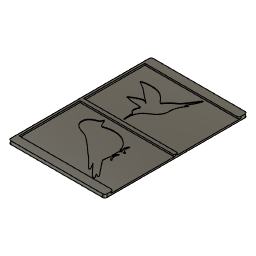
Wing Span - Lid (Autodesk Fusion 360 design; units mm, degrees)
Autodesk Fusion 360 part; units mm, degrees
note: some values were not read from the file. Set by a fixed rule: which sketch regions a step uses.
(part 1 of 2)
sketch "Skizze1" plane through (0, 0, 0) normal (0, 0, 1) x (1, 0, 0)
  line L0 (0, 0) -> (91.5, 0)
  line L1 (91.5, 0) -> (91.5, 135.5)
  line L2 (91.5, 135.5) -> (0, 135.5)
  line L3 (0, 135.5) -> (0, 0)
  line L4 (0, 0) -> (7, 0)
  line L5 (7, 0) -> (7, 7)
  line L6 (7, 7) -> (0, 7)
  line L7 (0, 7) -> (0, 0)
  line L8 (91.5, 0) -> (84.5, 0)
  line L9 (84.5, 0) -> (84.5, 7)
  line L10 (84.5, 7) -> (91.5, 7)
  line L11 (91.5, 7) -> (91.5, 0)
  line L12 (0, 135.5) -> (7, 135.5)
  line L13 (7, 135.5) -> (7, 128.5)
  line L14 (7, 128.5) -> (0, 128.5)
  line L15 (0, 128.5) -> (0, 135.5)
  line L16 (91.5, 135.5) -> (84.5, 135.5)
  line L17 (84.5, 135.5) -> (84.5, 128.5)
  line L18 (84.5, 128.5) -> (91.5, 128.5)
  line L19 (91.5, 128.5) -> (91.5, 135.5)
  circle A0 centre (3.5, 3.5) radius 2.675
  circle A1 centre (88, 3.5) radius 2.675
  circle A2 centre (88, 132) radius 2.675
  circle A3 centre (3.5, 132) radius 2.675
  dimension "d1" = 91.5
  dimension "d2" = 135.5
  dimension "d3" = 7
  dimension "d4" = 7
  dimension "d5" = 7
  dimension "d6" = 7
  dimension "d7" = 7
  dimension "d8" = 7
  dimension "d9" = 7
  dimension "d10" = 7
  dimension "d11" = 5.35
  dimension "d12" = 3.5
  dimension "d13" = 3.5
  dimension "d14" = 5.35
  dimension "d15" = 3.5
  dimension "d16" = 3.5
  dimension "d17" = 5.35
  dimension "d18" = 3.5
  dimension "d19" = 3.5
  dimension "d20" = 5.35
  dimension "d21" = 3.5
  dimension "d22" = 3.5
  constraint horizontal L0
  constraint vertical L1
  constraint horizontal L2
  constraint vertical L3
  constraint coincident L0.start L3.end
  constraint horizontal L4
  constraint vertical L5
  constraint horizontal L6
  constraint vertical L7
  constraint horizontal L8
  constraint vertical L9
  constraint horizontal L10
  constraint vertical L11
  constraint horizontal L12
  constraint vertical L13
  constraint horizontal L14
  constraint vertical L15
  constraint horizontal L16
  constraint vertical L17
  constraint horizontal L18
  constraint vertical L19
  measures "d1" distance of L0.start L0.end
  measures "d2" distance of L0.start L2.end
  measures "d3" distance of L0.start L4.end
  measures "d4" distance of L0.start L6.end
  measures "d5" distance of L0.end L8.end
  measures "d6" distance of L0.end L10.end
  measures "d7" distance of L2.end L12.end
  measures "d8" distance of L2.end L14.end
  measures "d9" distance of L1.end L16.end
  measures "d10" distance of L1.end L18.end
  measures "d11" diameter of A0
  measures "d12" distance of L4 A0.centre
  measures "d13" distance of L7 A0.centre
  measures "d14" diameter of A1
  measures "d15" distance of L11 A1.centre
  measures "d16" distance of L10 A1.centre
  measures "d17" diameter of A2
  measures "d18" distance of L19 A2.centre
  measures "d19" distance of L2 A2.centre
  measures "d20" diameter of A3
  measures "d21" distance of L12 A3.centre
  measures "d22" distance of L13 A3.centre
extrude "Extrusion6" add sketch "Skizze1" along normal blind 3 contours L0 L3 L4 L5 L6 L7 | L0 L1 L2 L3 L5 L6 L9 L10 L13 L14 L17 L18 | L0 L1 L8 L9 L10 L11 | L2 L3 L12 L13 L14 L15 | L1 L2 L16 L17 L18 L19 | A0 | A1 | A2 | A3 picked at (3.433366, 0.277493) picked at (58.666667, 47.5) picked at (87.933366, 0.277493) picked at (3.433366, 128.777493) picked at (88.066634, 128.777493) picked at (2.696636, 4.326095) picked at (88.803364, 3.621088) picked at (88.700923, 133.066531) picked at (1.893588, 131.564999)
extrude "Extrusion7" cut sketch "Skizze1" along normal blind 1.2 contours A0 | A1 | A2 | A3 picked at (2.696636, 4.326095) picked at (88.803364, 3.621088) picked at (88.700923, 133.066531) picked at (1.893588, 131.564999)
sketch "Skizze6" plane through (0, 0, 3) normal (0, 0, 1) x (-1, 0, 0)
  line L0 (-91.5, 0) -> (-91.5, -135.5)
  line L1 (-91.5, -135.5) -> (0, -135.5)
  line L2 (0, -135.5) -> (0, 0)
  line L3 (0, 0) -> (-91.5, 0)
  line L4 (-2, -8) -> (-91.5, -8)
  line L5 (-91.5, -8) -> (-91.5, -66)
  line L6 (-91.5, -66) -> (-2, -66)
  line L7 (-2, -66) -> (-2, -8)
  line L8 (-2, -69.499999) -> (-91.5, -69.499999)
  line L9 (-91.5, -69.499999) -> (-91.5, -127.5)
  line L10 (-91.5, -127.5) -> (-2, -127.5)
  line L11 (-2, -127.5) -> (-2, -69.499999)
  dimension "d51" = 89.5
  dimension "d52" = 58
  dimension "d53" = 2
  dimension "d54" = 8
  dimension "d55" = 2
  dimension "d56" = 58
  dimension "d57" = 8
  dimension "d58" = 89.5
  constraint horizontal L4
  constraint vertical L5
  constraint horizontal L6
  constraint vertical L7
  constraint horizontal L8
  constraint vertical L9
  constraint horizontal L10
  constraint vertical L11
  measures "d51" distance of L4.start L4.end
  measures "d52" distance of L4.start L6.end
  measures "d53" distance of L2 L7
  measures "d54" distance of L3 L4
  measures "d55" distance of L2 L11
  measures "d56" distance of L8 L10
  measures "d57" distance of L1 L10
  measures "d58" distance of L9 L11
extrude "Extrusion9" cut sketch "Skizze6" against normal blind 1.5 contours L0 L4 L5 L6 L7 | L0 L8 L9 L10 L11 picked at (-61.666667, -27.333333) picked at (-61.666667, -88.833333)
fillet "Abrundung3" radius 2 2 edges at (0, 0, 1.5) (0, 135.5, 1.5)
fillet "Abrundung4" radius 1 1 edges at (91.5, 66, 2.25)
fillet "Abrundung5" radius 1 1 edges at (91.5, 69.499999, 2.25)
fillet "Abrundung6" radius 2 1 edges at (91.5, 8, 2.25)
fillet "Abrundung7" radius 2 1 edges at (91.5, 127.5, 2.25)
fillet "Abrundung8" radius 2 2 edges at (91.5, 135.5, 1.5) (91.5, 0, 1.5)
sketch "Skizze7" plane through (0, 0, 1.5) normal (0, 0, 1) x (-1, 0, 0)
  line L0 (-2, -66) -> (-2, -8)
  line L1 (-2, -8) -> (-89.5, -8)
  arc A0 (-91.5, -6) -> (-89.5, -8) centre (-89.5, -6) ccw
  line L2 (-91.5, -6) -> (-91.5, -67)
  arc A1 (-90.5, -66) -> (-91.5, -67) centre (-90.5, -67) ccw
  line L3 (-90.5, -66) -> (-2, -66)
  spline S0 degree 3 poles (-30.411065, -58.609692) (-28.836348, -62.212151) (-28.526911, -62.854914) (-28.162708, -62.873627) knots 0 0 0 0 1 1 1 1
  spline S1 degree 3 poles (-28.162708, -62.873627) (-28.080965, -62.877743) (-27.963864, -62.847698) (-27.869518, -62.680787) knots 0 0 0 0 1 1 1 1
  spline S2 degree 3 poles (-27.869518, -62.680787) (-27.684016, -62.352588) (-27.563036, -62.031554) (-27.446005, -61.720969) knots 0 0 0 0 1 1 1 1
  spline S3 degree 3 poles (-27.446005, -61.720969) (-27.205823, -61.083809) (-26.998358, -60.533474) (-26.308111, -60.053195) knots 0 0 0 0 1 1 1 1
  spline S4 degree 3 poles (-26.308111, -60.053195) (-25.982101, -59.826301) (-25.405463, -59.594364) (-24.737778, -59.325714) knots 0 0 0 0 1 1 1 1
  spline S5 degree 3 poles (-24.737778, -59.325714) (-22.624632, -58.475447) (-19.431234, -57.190489) (-18.33478, -53.917152) knots 0 0 0 0 1 1 1 1
  spline S6 degree 3 poles (-18.33478, -53.917152) (-18.152793, -53.372845) (-18.035865, -52.81678) (-17.987487, -52.263824) knots 0 0 0 0 1 1 1 1
  spline S7 degree 3 poles (-17.987487, -52.263824) (-17.808073, -50.213115) (-18.547131, -48.264464) (-20.124662, -46.628865) knots 0 0 0 0 1 1 1 1
  spline S8 degree 3 poles (-20.124662, -46.628865) (-21.885668, -44.80306) (-24.550983, -43.48011) (-28.046934, -42.69664) knots 0 0 0 0 1 1 1 1
  spline S9 degree 3 poles (-28.046934, -42.69664) (-32.434766, -41.713249) (-40.268695, -34.518616) (-44.949472, -30.220073) knots 0 0 0 0 1 1 1 1
  spline S10 degree 3 poles (-44.949472, -30.220073) (-46.538387, -28.760833) (-47.793338, -27.608143) (-48.426302, -27.148487) knots 0 0 0 0 1 1 1 1
  spline S11 degree 3 poles (-48.426302, -27.148487) (-50.763295, -25.450827) (-53.762076, -22.368466) (-56.171671, -19.891637) knots 0 0 0 0 1 1 1 1
  spline S12 degree 3 poles (-56.171671, -19.891637) (-58.950819, -17.035183) (-60.429083, -15.544488) (-61.031372, -15.547429) knots 0 0 0 0 1 1 1 1
  spline S13 degree 3 poles (-61.031372, -15.547429) (-61.150111, -15.547999) (-61.224441, -15.599828) (-61.265834, -15.643243) knots 0 0 0 0 1 1 1 1
  spline S14 degree 3 poles (-61.265834, -15.643243) (-61.323003, -15.703148) (-61.356462, -15.785022) (-61.365362, -15.886746) knots 0 0 0 0 1 1 1 1
  spline S15 degree 3 poles (-61.365362, -15.886746) (-61.437672, -16.713253) (-59.650855, -19.65266) (-57.870181, -22.384839) knots 0 0 0 0 1 1 1 1
  spline S16 degree 3 poles (-57.870181, -22.384839) (-59.546777, -20.484485) (-61.836065, -18.04111) (-64.07326, -15.653713) knots 0 0 0 0 1 1 1 1
  spline S17 degree 3 poles (-64.07326, -15.653713) (-64.765743, -14.914723) (-65.44634, -14.188238) (-66.091815, -13.495845) knots 0 0 0 0 1 1 1 1
  spline S18 degree 3 poles (-66.091815, -13.495845) (-68.098082, -11.343941) (-69.849858, -10.110189) (-70.554899, -10.352979) knots 0 0 0 0 1 1 1 1
  spline S19 degree 3 poles (-70.554899, -10.352979) (-70.7336, -10.414559) (-70.842148, -10.562693) (-70.860284, -10.769989) knots 0 0 0 0 1 1 1 1
  spline S20 degree 3 poles (-70.860284, -10.769989) (-70.909057, -11.327464) (-70.309448, -12.235853) (-69.797711, -12.899855) knots 0 0 0 0 1 1 1 1
  spline S21 degree 3 poles (-69.797711, -12.899855) (-68.87248, -14.100238) (-68.549162, -14.7867) (-68.552585, -15.037768) knots 0 0 0 0 1 1 1 1
  spline S22 degree 3 poles (-68.552585, -15.037768) (-68.62865, -15.030438) (-68.844737, -14.948986) (-69.247923, -14.618512) knots 0 0 0 0 1 1 1 1
  spline S23 degree 3 poles (-69.247923, -14.618512) (-70.158248, -13.872096) (-70.957131, -13.534144) (-71.384918, -13.714199) knots 0 0 0 0 1 1 1 1
  spline S24 degree 3 poles (-71.384918, -13.714199) (-71.554173, -13.785372) (-71.656843, -13.931829) (-71.673866, -14.12641) knots 0 0 0 0 1 1 1 1
  spline S25 degree 3 poles (-71.673866, -14.12641) (-71.709714, -14.53615) (-71.359214, -15.158565) (-70.687885, -15.879183) knots 0 0 0 0 1 1 1 1
  spline S26 degree 3 poles (-70.687885, -15.879183) (-68.877183, -17.822964) (-63.804399, -24.350677) (-61.366924, -27.487781) knots 0 0 0 0 1 1 1 1
  spline S27 degree 3 poles (-61.366924, -27.487781) (-60.691105, -28.357487) (-60.235951, -28.941854) (-60.116939, -29.086464) knots 0 0 0 0 1 1 1 1
  spline S28 degree 3 poles (-60.116939, -29.086464) (-60.10674, -29.125964) (-60.090835, -29.260204) (-60.130401, -29.712441) knots 0 0 0 0 1 1 1 1
  spline S29 degree 3 poles (-60.130401, -29.712441) (-60.161096, -30.063288) (-60.211755, -30.540179) (-60.276205, -31.091899) knots 0 0 0 0 1 1 1 1
  spline S30 degree 3 poles (-60.276205, -31.091899) (-60.375065, -31.936651) (-60.487675, -32.988745) (-60.591881, -34.17982) knots 0 0 0 0 1 1 1 1
  spline S31 degree 3 poles (-60.591881, -34.17982) (-60.591925, -34.180323) (-60.591925, -34.180323) (-60.591969, -34.180823) knots 0 0 0 0 1 1 1 1
  spline S32 degree 3 poles (-60.591969, -34.180823) (-60.641254, -34.744154) (-60.681431, -35.29395) (-60.714118, -35.833276) knots 0 0 0 0 1 1 1 1
  spline S33 degree 3 poles (-60.714118, -35.833276) (-61.229939, -35.813268) (-61.848921, -35.717977) (-61.968396, -35.524606) knots 0 0 0 0 1 1 1 1
  spline S34 degree 3 poles (-61.968396, -35.524606) (-61.979314, -35.506791) (-61.992581, -35.481186) (-62.010059, -35.447792) knots 0 0 0 0 1 1 1 1
  spline S35 degree 3 poles (-62.010059, -35.447792) (-62.125041, -35.228176) (-62.394615, -34.713657) (-63.17529, -33.893952) knots 0 0 0 0 1 1 1 1
  spline S36 degree 3 poles (-63.17529, -33.893952) (-63.488116, -33.565483) (-63.922238, -33.195547) (-64.214248, -33.297792) knots 0 0 0 0 1 1 1 1
  spline S37 degree 3 poles (-64.214248, -33.297792) (-64.3193, -33.334626) (-64.388048, -33.42673) (-64.398338, -33.544349) knots 0 0 0 0 1 1 1 1
  spline S38 degree 3 poles (-64.398338, -33.544349) (-64.410751, -33.686229) (-64.338206, -33.864872) (-64.194145, -34.04691) knots 0 0 0 0 1 1 1 1
  spline S39 degree 3 poles (-64.194145, -34.04691) (-63.145869, -35.372868) (-62.620912, -37.005394) (-62.75394, -38.525902) knots 0 0 0 0 1 1 1 1
  spline S40 degree 3 poles (-62.75394, -38.525902) (-62.774066, -38.755952) (-62.809751, -38.984641) (-62.859956, -39.205821) knots 0 0 0 0 1 1 1 1
  spline S41 degree 3 poles (-62.859956, -39.205821) (-63.089233, -40.215509) (-63.184234, -40.391803) (-63.356533, -40.711717) knots 0 0 0 0 1 1 1 1
  spline S42 degree 3 poles (-63.356533, -40.711717) (-63.435424, -40.858063) (-63.53329, -41.040175) (-63.664042, -41.339954) knots 0 0 0 0 1 1 1 1
  spline S43 degree 3 poles (-63.664042, -41.339954) (-63.722522, -41.474598) (-63.66048, -41.605627) (-63.534094, -41.640961) knots 0 0 0 0 1 1 1 1
  spline S44 degree 3 poles (-63.534094, -41.640961) (-63.230795, -41.725659) (-62.323651, -41.165393) (-62.076992, -40.664177) knots 0 0 0 0 1 1 1 1
  spline S45 degree 3 poles (-62.076992, -40.664177) (-61.851467, -40.206124) (-61.711742, -39.682401) (-61.661491, -39.108029) knots 0 0 0 0 1 1 1 1
  spline S46 degree 3 poles (-61.661491, -39.108029) (-61.609029, -38.508393) (-61.660517, -37.969626) (-61.698255, -37.576208) knots 0 0 0 0 1 1 1 1
  spline S47 degree 3 poles (-61.698255, -37.576208) (-61.715564, -37.396326) (-61.730574, -37.238393) (-61.727735, -37.142377) knots 0 0 0 0 1 1 1 1
  spline S48 degree 3 poles (-61.727735, -37.142377) (-61.507514, -37.147652) (-61.084822, -37.191542) (-60.781233, -37.226703) knots 0 0 0 0 1 1 1 1
  spline S49 degree 3 poles (-60.781233, -37.226703) (-60.859949, -39.48111) (-60.781837, -41.511529) (-60.543162, -43.325362) knots 0 0 0 0 1 1 1 1
  spline S50 degree 3 poles (-60.543162, -43.325362) (-61.408855, -44.516069) (-62.226714, -45.612845) (-62.365345, -45.719402) knots 0 0 0 0 1 1 1 1
  spline S51 degree 3 poles (-62.365345, -45.719402) (-62.446011, -45.768484) (-62.78663, -45.645961) (-63.035391, -45.556423) knots 0 0 0 0 1 1 1 1
  spline S52 degree 3 poles (-63.035391, -45.556423) (-63.344135, -45.445287) (-63.693918, -45.319598) (-64.066381, -45.264253) knots 0 0 0 0 1 1 1 1
  spline S53 degree 3 poles (-64.066381, -45.264253) (-64.56832, -45.189655) (-65.015577, -45.328218) (-65.218583, -45.488489) knots 0 0 0 0 1 1 1 1
  spline S54 degree 3 poles (-65.218583, -45.488489) (-65.309499, -45.560279) (-65.359299, -45.640047) (-65.366793, -45.725708) knots 0 0 0 0 1 1 1 1
  spline S55 degree 3 poles (-65.366793, -45.725708) (-65.37199, -45.785102) (-65.363625, -45.98241) (-65.037091, -46.030873) knots 0 0 0 0 1 1 1 1
  spline S56 degree 3 poles (-65.037091, -46.030873) (-64.55744, -46.102004) (-63.091419, -46.923336) (-62.63891, -47.505111) knots 0 0 0 0 1 1 1 1
  spline S57 degree 3 poles (-62.63891, -47.505111) (-61.901221, -48.453903) (-61.892346, -49.219572) (-62.035033, -50.357209) knots 0 0 0 0 1 1 1 1
  spline S58 degree 3 poles (-62.035033, -50.357209) (-62.150078, -51.275232) (-62.446662, -51.951966) (-62.589245, -52.277176) knots 0 0 0 0 1 1 1 1
  spline S59 degree 3 poles (-62.589245, -52.277176) (-62.65073, -52.41729) (-62.678748, -52.481261) (-62.683681, -52.537645) knots 0 0 0 0 1 1 1 1
  spline S60 degree 3 poles (-62.683681, -52.537645) (-62.689566, -52.604904) (-62.661621, -52.667031) (-62.608855, -52.70368) knots 0 0 0 0 1 1 1 1
  line L4 (-62.608855, -52.70368) -> (-62.513581, -52.757368)
  line L5 (-62.513581, -52.757368) -> (-62.425652, -52.715834)
  spline S61 degree 3 poles (-62.425652, -52.715834) (-62.219039, -52.618426) (-61.372342, -52.053376) (-61.00616, -51.068652) knots 0 0 0 0 1 1 1 1
  spline S62 degree 3 poles (-61.00616, -51.068652) (-60.794757, -50.500288) (-60.665915, -49.964148) (-60.623158, -49.475437) knots 0 0 0 0 1 1 1 1
  spline S63 degree 3 poles (-60.623158, -49.475437) (-60.540806, -48.534154) (-60.780273, -47.939492) (-60.955042, -47.505259) knots 0 0 0 0 1 1 1 1
  spline S64 degree 3 poles (-60.955042, -47.505259) (-61.051467, -47.266192) (-61.126128, -47.090564) (-61.088861, -46.959458) knots 0 0 0 0 1 1 1 1
  spline S65 degree 3 poles (-61.088861, -46.959458) (-61.034125, -46.769356) (-60.656316, -46.187396) (-60.16179, -45.479593) knots 0 0 0 0 1 1 1 1
  spline S66 degree 3 poles (-60.16179, -45.479593) (-59.628284, -47.825667) (-58.764628, -49.735652) (-57.563723, -51.236304) knots 0 0 0 0 1 1 1 1
  spline S67 degree 3 poles (-57.563723, -51.236304) (-51.483372, -58.83454) (-43.256991, -59.209826) (-37.417781, -58.187366) knots 0 0 0 0 1 1 1 1
  spline S68 degree 3 poles (-37.417781, -58.187366) (-35.827556, -57.908898) (-34.653983, -57.471239) (-33.797253, -57.151863) knots 0 0 0 0 1 1 1 1
  spline S69 degree 3 poles (-33.797253, -57.151863) (-31.981501, -56.474841) (-31.433584, -56.270567) (-30.411065, -58.609692) knots 0 0 0 0 1 1 1 1
  spline S70 degree 3 poles (-36.593582, -73.055306) (-36.449055, -73.033535) (-36.40256, -73.207057) (-36.374795, -73.31068) knots 0 0 0 0 1 1 1 1
  spline S71 degree 3 poles (-36.374795, -73.31068) (-36.152736, -74.139413) (-35.748667, -78.071569) (-35.91474, -81.444122) knots 0 0 0 0 1 1 1 1
  spline S72 degree 3 poles (-35.91474, -81.444122) (-35.925543, -81.662306) (-35.914713, -81.828298) (-35.88169, -81.951542) knots 0 0 0 0 1 1 1 1
  spline S73 degree 3 poles (-35.88169, -81.951542) (-35.817254, -82.192019) (-35.678448, -82.254846) (-35.370463, -82.373681) knots 0 0 0 0 1 1 1 1
  spline S74 degree 3 poles (-35.370463, -82.373681) (-34.999119, -82.517069) (-34.490673, -82.713493) (-33.910176, -83.451048) knots 0 0 0 0 1 1 1 1
  spline S75 degree 3 poles (-33.910176, -83.451048) (-33.67064, -83.755405) (-33.488946, -84.134279) (-33.370327, -84.576972) knots 0 0 0 0 1 1 1 1
  spline S76 degree 3 poles (-33.370327, -84.576972) (-32.903045, -86.320894) (-33.454243, -88.831515) (-34.680928, -90.546836) knots 0 0 0 0 1 1 1 1
  spline S77 degree 3 poles (-34.680928, -90.546836) (-34.68857, -90.557558) (-34.689316, -90.562621) (-34.689185, -90.563112) knots 0 0 0 0 1 1 1 1
  spline S78 degree 3 poles (-34.689185, -90.563112) (-34.659185, -90.675072) (-34.117772, -90.947438) (-32.282185, -91.176905) knots 0 0 0 0 1 1 1 1
  spline S79 degree 3 poles (-32.282185, -91.176905) (-30.939964, -91.344705) (-29.271859, -91.439642) (-28.032254, -91.418727) knots 0 0 0 0 1 1 1 1
  spline S80 degree 3 poles (-28.032254, -91.418727) (-26.17269, -91.387444) (-23.382909, -91.996986) (-21.537005, -92.400336) knots 0 0 0 0 1 1 1 1
  spline S81 degree 3 poles (-21.537005, -92.400336) (-20.749344, -92.572414) (-20.127231, -92.708414) (-19.895075, -92.722307) knots 0 0 0 0 1 1 1 1
  spline S82 degree 3 poles (-19.895075, -92.722307) (-19.716185, -92.733126) (-19.609698, -92.79699) (-19.578777, -92.912386) knots 0 0 0 0 1 1 1 1
  spline S83 degree 3 poles (-19.578777, -92.912386) (-19.558931, -92.986455) (-19.576662, -93.067438) (-19.632971, -93.159939) knots 0 0 0 0 1 1 1 1
  spline S84 degree 3 poles (-19.632971, -93.159939) (-20.270523, -94.205862) (-26.968935, -97.78965) (-29.189433, -98.272649) knots 0 0 0 0 1 1 1 1
  spline S85 degree 3 poles (-29.189433, -98.272649) (-31.012855, -98.66936) (-32.611223, -97.574054) (-33.379313, -97.047775) knots 0 0 0 0 1 1 1 1
  spline S86 degree 3 poles (-33.379313, -97.047775) (-33.470131, -96.985494) (-33.567209, -96.918975) (-33.646898, -96.868303) knots 0 0 0 0 1 1 1 1
  spline S87 degree 3 poles (-33.646898, -96.868303) (-33.419517, -97.196949) (-32.592971, -97.79129) (-31.496344, -98.579813) knots 0 0 0 0 1 1 1 1
  spline S88 degree 3 poles (-31.496344, -98.579813) (-29.914233, -99.71746) (-27.523435, -101.436753) (-24.756233, -103.891244) knots 0 0 0 0 1 1 1 1
  spline S89 degree 3 poles (-24.756233, -103.891244) (-20.879724, -107.32972) (-17.429784, -109.273341) (-15.36871, -110.434589) knots 0 0 0 0 1 1 1 1
  spline S90 degree 3 poles (-15.36871, -110.434589) (-13.995973, -111.208271) (-13.435482, -111.534669) (-13.351791, -111.847008) knots 0 0 0 0 1 1 1 1
  spline S91 degree 3 poles (-13.351791, -111.847008) (-13.331912, -111.921199) (-13.323539, -112.063796) (-13.491542, -112.183861) knots 0 0 0 0 1 1 1 1
  spline S92 degree 3 poles (-13.491542, -112.183861) (-14.351732, -112.798663) (-24.35914, -114.996724) (-30.897149, -111.974879) knots 0 0 0 0 1 1 1 1
  spline S93 degree 3 poles (-30.897149, -111.974879) (-34.54769, -110.28768) (-36.929454, -107.52737) (-38.50557, -105.700846) knots 0 0 0 0 1 1 1 1
  spline S94 degree 3 poles (-38.50557, -105.700846) (-39.413733, -104.648375) (-40.131093, -103.816981) (-40.60366, -103.785356) knots 0 0 0 0 1 1 1 1
  spline S95 degree 3 poles (-40.60366, -103.785356) (-40.711102, -103.778264) (-40.803227, -103.812149) (-40.893711, -103.892386) knots 0 0 0 0 1 1 1 1
  spline S96 degree 3 poles (-40.893711, -103.892386) (-41.237589, -104.197321) (-41.629928, -104.673092) (-42.126811, -105.275716) knots 0 0 0 0 1 1 1 1
  spline S97 degree 3 poles (-42.126811, -105.275716) (-43.494054, -106.933937) (-45.560388, -109.439805) (-49.461074, -111.914077) knots 0 0 0 0 1 1 1 1
  spline S98 degree 3 poles (-49.461074, -111.914077) (-51.213679, -113.025875) (-56.237332, -121.085237) (-57.429859, -123.150748) knots 0 0 0 0 1 1 1 1
  spline S99 degree 3 poles (-57.429859, -123.150748) (-57.488032, -123.251505) (-58.861049, -125.617076) (-59.44855, -125.539623) knots 0 0 0 0 1 1 1 1
  spline S100 degree 3 poles (-59.44855, -125.539623) (-59.4954, -125.533513) (-59.608859, -125.502009) (-59.651411, -125.343203) knots 0 0 0 0 1 1 1 1
  spline S101 degree 3 poles (-59.651411, -125.343203) (-59.75577, -124.95373) (-59.363708, -123.747519) (-58.483662, -121.757325) knots 0 0 0 0 1 1 1 1
  spline S102 degree 3 poles (-58.483662, -121.757325) (-57.33193, -119.152559) (-56.279933, -117.302796) (-55.511055, -115.95185) knots 0 0 0 0 1 1 1 1
  spline S103 degree 3 poles (-55.511055, -115.95185) (-54.762695, -114.637158) (-54.296699, -113.814773) (-54.347117, -113.349466) knots 0 0 0 0 1 1 1 1
  spline S104 degree 3 poles (-54.347117, -113.349466) (-54.554947, -113.448921) (-55.082394, -113.728519) (-56.395021, -114.499644) knots 0 0 0 0 1 1 1 1
  spline S105 degree 3 poles (-56.395021, -114.499644) (-56.426704, -114.518255) (-56.502226, -114.559651) (-56.573083, -114.530664) knots 0 0 0 0 1 1 1 1
  line L6 (-56.573083, -114.530664) -> (-56.655382, -114.506056)
  line L7 (-56.655382, -114.506056) -> (-56.671647, -114.445354)
  spline S106 degree 3 poles (-56.671647, -114.445354) (-56.67168, -114.445231) (-56.671713, -114.445109) (-56.671745, -114.444986) knots 0 0 0 0 1 1 1 1
  spline S107 degree 3 poles (-56.671745, -114.444986) (-56.697145, -114.350193) (-56.634469, -114.280957) (-56.233686, -113.732211) knots 0 0 0 0 1 1 1 1
  spline S108 degree 3 poles (-56.233686, -113.732211) (-55.011173, -112.058225) (-51.271665, -106.959021) (-51.651519, -101.369032) knots 0 0 0 0 1 1 1 1
  spline S109 degree 3 poles (-51.651519, -101.369032) (-51.87403, -98.093373) (-50.023429, -93.456007) (-46.05575, -90.931057) knots 0 0 0 0 1 1 1 1
  spline S110 degree 3 poles (-46.05575, -90.931057) (-40.055273, -87.112245) (-36.395469, -84.281005) (-36.748233, -74.613367) knots 0 0 0 0 1 1 1 1
  spline S111 degree 3 poles (-36.748233, -74.613367) (-36.803817, -73.086926) (-36.720204, -73.074249) (-36.593582, -73.055306) knots 0 0 0 0 1 1 1 1
extrude "Extrusion10" cut sketch "Skizze7" against normal blind 0.5 contours S0 S1 S2 S3 S4 S5 S6 S7 S8 S9 S10 S11 S12 S13 S14 S15 S16 S17 S18 S19 S20 S21 S22 S23 S24 S25 S26 S27 S28 S29 S30 S32 S33 S34 S35 S36 S37 S38 S39 S40 S41 S42 S43 S44 S45 S46 S47 S48 S49 S50 S51 S52 S53 S54 S55 S56 S57 S58 S59 S60 L4 L5 S61 S62 S63 S64 S65 S66 S67 S68 S69 | S70 S71 S72 S73 S74 S75 S76 S77 S78 S79 S80 S81 S82 S83 S84 S85 S86 S87 S88 S89 S90 S91 S92 S93 S94 S95 S96 S97 S98 S99 S100 S101 S102 S103 S104 S105 L6 L7 S107 S108 S109 S110 S111 picked at (-47.757365, -36.705446) picked at (-40.102103, -97.194906)
sketch "Skizze5" plane through (0, 0, 3) normal (0, 0, 1) x (-1, 0, 0)
  line L0 (-91.5, 0) -> (-91.5, -135.5)
  line L1 (-91.5, -135.5) -> (0, -135.5)
  line L2 (0, -135.5) -> (0, 0)
  line L3 (0, 0) -> (-91.5, 0)
extrude "Extrusion1" [suppressed]
extrude "Extrusion2" [suppressed]
sketch "Skizze2" plane through (0, 0, 3) normal (0, 0, 1) x (-1, 0, 0)
  line L0 (-91.5, 0) -> (-91.5, -135.5)
  line L1 (-91.5, -135.5) -> (0, -135.5)
  line L2 (0, -135.5) -> (0, 0)
  line L3 (0, 0) -> (-91.5, 0)
  line L4 (-2, -5) -> (-91.5, -5)
  line L5 (-91.5, -5) -> (-91.5, -63)
  line L6 (-91.5, -63) -> (-2, -63)
  line L7 (-2, -63) -> (-2, -5)
  line L8 (-2, -72.5) -> (-91.5, -72.5)
  line L9 (-91.5, -72.5) -> (-91.5, -130.5)
  line L10 (-91.5, -130.5) -> (-2, -130.5)
  line L11 (-2, -130.5) -> (-2, -72.5)
  dimension "d27" = 58
  dimension "d28" = 89.5
  dimension "d29" = 2
  dimension "d30" = 2
  dimension "d31" = 58
  dimension "d32" = 89.5
  dimension "d33" = 5
  dimension "d34" = 5
  constraint horizontal L4
  constraint vertical L5
  constraint horizontal L6
  constraint vertical L7
  constraint horizontal L8
  constraint vertical L9
  constraint horizontal L10
  constraint vertical L11
  measures "d27" distance of L4 L6
  measures "d28" distance of L5 L7
  measures "d29" distance of L2 L7
  measures "d30" distance of L2 L11
  measures "d31" distance of L8 L10
  measures "d32" distance of L9 L11
  measures "d33" distance of L3 L4
  measures "d34" distance of L1 L10
extrude "Extrusion3" [suppressed]
fillet "Abrundung1" [suppressed]
fillet "Abrundung2" [suppressed]
sketch "Skizze3" plane through (0, 0, 1.75) normal (0, 0, 1) x (-1, 0, 0)
  line L0 (-2, -63) -> (-2, -5)
  line L1 (-2, -5) -> (-91.5, -5)
  line L2 (-91.5, -5) -> (-91.5, -63)
  line L3 (-91.5, -63) -> (-2, -63)
  spline S0 degree 3 poles (-31.274079, -52.30811) (-29.378628, -55.782991) (-29.011881, -56.400493) (-28.644965, -56.387304) knots 0 0 0 0 1 1 1 1
  spline S1 degree 3 poles (-28.644965, -56.387304) (-28.56262, -56.384259) (-28.44781, -56.343851) (-28.367833, -56.16817) knots 0 0 0 0 1 1 1 1
  spline S2 degree 3 poles (-28.367833, -56.16817) (-28.210583, -55.822728) (-28.117417, -55.490135) (-28.027294, -55.168367) knots 0 0 0 0 1 1 1 1
  spline S3 degree 3 poles (-28.027294, -55.168367) (-27.842314, -54.508258) (-27.682528, -53.938099) (-27.032394, -53.395841) knots 0 0 0 0 1 1 1 1
  spline S4 degree 3 poles (-27.032394, -53.395841) (-26.725334, -53.139674) (-26.167351, -52.856457) (-25.521274, -52.52843) knots 0 0 0 0 1 1 1 1
  spline S5 degree 3 poles (-25.521274, -52.52843) (-23.47652, -51.490241) (-20.386478, -49.921296) (-19.574021, -46.542119) knots 0 0 0 0 1 1 1 1
  spline S6 degree 3 poles (-19.574021, -46.542119) (-19.439259, -45.980243) (-19.370779, -45.412282) (-19.370779, -44.853455) knots 0 0 0 0 1 1 1 1
  spline S7 degree 3 poles (-19.370779, -44.853455) (-19.370779, -42.78097) (-20.282997, -40.891436) (-22.008686, -39.389448) knots 0 0 0 0 1 1 1 1
  spline S8 degree 3 poles (-22.008686, -39.389448) (-23.93508, -37.712794) (-26.724319, -36.619822) (-30.2993, -36.140804) knots 0 0 0 0 1 1 1 1
  spline S9 degree 3 poles (-30.2993, -36.140804) (-34.786329, -35.539535) (-43.274603, -29.011133) (-48.346329, -25.110664) knots 0 0 0 0 1 1 1 1
  spline S10 degree 3 poles (-48.346329, -25.110664) (-50.067962, -23.786554) (-51.427748, -22.740589) (-52.102907, -22.335121) knots 0 0 0 0 1 1 1 1
  spline S11 degree 3 poles (-52.102907, -22.335121) (-54.595737, -20.837528) (-57.873805, -18.009231) (-60.50782, -15.736549) knots 0 0 0 0 1 1 1 1
  spline S12 degree 3 poles (-60.50782, -15.736549) (-63.545786, -13.115551) (-65.159201, -11.750183) (-65.763004, -11.805981) knots 0 0 0 0 1 1 1 1
  spline S13 degree 3 poles (-65.763004, -11.805981) (-65.882042, -11.816972) (-65.952043, -11.875475) (-65.989748, -11.92265) knots 0 0 0 0 1 1 1 1
  spline S14 degree 3 poles (-65.989748, -11.92265) (-66.041829, -11.987748) (-66.068202, -12.072799) (-66.068202, -12.175602) knots 0 0 0 0 1 1 1 1
  spline S15 degree 3 poles (-66.068202, -12.175602) (-66.068202, -13.010886) (-64.018208, -15.802153) (-61.992558, -18.386123) knots 0 0 0 0 1 1 1 1
  spline S16 degree 3 poles (-61.992558, -18.386123) (-63.840835, -16.627293) (-66.351254, -14.377607) (-68.804514, -12.179492) knots 0 0 0 0 1 1 1 1
  spline S17 degree 3 poles (-68.804514, -12.179492) (-69.563878, -11.49909) (-70.310223, -10.830187) (-71.018352, -10.192396) knots 0 0 0 0 1 1 1 1
  spline S18 degree 3 poles (-71.018352, -10.192396) (-73.219341, -8.210204) (-75.084527, -7.126533) (-75.770339, -7.431902) knots 0 0 0 0 1 1 1 1
  spline S19 degree 3 poles (-75.770339, -7.431902) (-75.944161, -7.509343) (-76.040031, -7.667438) (-76.040031, -7.876936) knots 0 0 0 0 1 1 1 1
  spline S20 degree 3 poles (-76.040031, -7.876936) (-76.040031, -8.44033) (-75.358951, -9.298778) (-74.787445, -9.91983) knots 0 0 0 0 1 1 1 1
  spline S21 degree 3 poles (-74.787445, -9.91983) (-73.754163, -11.042559) (-73.369659, -11.70267) (-73.351063, -11.954777) knots 0 0 0 0 1 1 1 1
  spline S22 degree 3 poles (-73.351063, -11.954777) (-73.427994, -11.9541) (-73.651865, -11.89137) (-74.085235, -11.595301) knots 0 0 0 0 1 1 1 1
  spline S23 degree 3 poles (-74.085235, -11.595301) (-75.063732, -10.926567) (-75.894619, -10.65772) (-76.307865, -10.875841) knots 0 0 0 0 1 1 1 1
  spline S24 degree 3 poles (-76.307865, -10.875841) (-76.471373, -10.962074) (-76.561494, -11.117971) (-76.561494, -11.314618) knots 0 0 0 0 1 1 1 1
  spline S25 degree 3 poles (-76.561494, -11.314618) (-76.561494, -11.72871) (-76.155348, -12.3222) (-75.418813, -12.986032) knots 0 0 0 0 1 1 1 1
  spline S26 degree 3 poles (-75.418813, -12.986032) (-73.432226, -14.776649) (-67.771738, -20.878448) (-65.051825, -23.810901) knots 0 0 0 0 1 1 1 1
  spline S27 degree 3 poles (-65.051825, -23.810901) (-64.297704, -24.623865) (-63.789936, -25.170013) (-63.657884, -25.304606) knots 0 0 0 0 1 1 1 1
  spline S28 degree 3 poles (-63.657884, -25.304606) (-63.644189, -25.343328) (-63.616459, -25.476566) (-63.616459, -25.933605) knots 0 0 0 0 1 1 1 1
  spline S29 degree 3 poles (-63.616459, -25.933605) (-63.616459, -26.288178) (-63.625422, -26.770917) (-63.64165, -27.329915) knots 0 0 0 0 1 1 1 1
  spline S30 degree 3 poles (-63.64165, -27.329915) (-63.666677, -28.185826) (-63.687301, -29.250897) (-63.687301, -30.454619) knots 0 0 0 0 1 1 1 1
  spline S31 degree 3 poles (-63.687301, -30.454619) (-63.687301, -30.455127) (-63.687301, -30.455127) (-63.687301, -30.455633) knots 0 0 0 0 1 1 1 1
  spline S32 degree 3 poles (-63.687301, -30.455633) (-63.687301, -31.024946) (-63.679355, -31.579885) (-63.664814, -32.123665) knots 0 0 0 0 1 1 1 1
  spline S33 degree 3 poles (-63.664814, -32.123665) (-64.183908, -32.148859) (-64.813073, -32.107602) (-64.949867, -31.924145) knots 0 0 0 0 1 1 1 1
  spline S34 degree 3 poles (-64.949867, -31.924145) (-64.96238, -31.907235) (-64.977932, -31.88272) (-64.998392, -31.850761) knots 0 0 0 0 1 1 1 1
  spline S35 degree 3 poles (-64.998392, -31.850761) (-65.132983, -31.640588) (-65.448496, -31.14821) (-66.303394, -30.394594) knots 0 0 0 0 1 1 1 1
  spline S36 degree 3 poles (-66.303394, -30.394594) (-66.645962, -30.092608) (-67.113822, -29.759676) (-67.397719, -29.887845) knots 0 0 0 0 1 1 1 1
  spline S37 degree 3 poles (-67.397719, -29.887845) (-67.499848, -29.934005) (-67.560716, -30.032413) (-67.560716, -30.151281) knots 0 0 0 0 1 1 1 1
  spline S38 degree 3 poles (-67.560716, -30.151281) (-67.560716, -30.294667) (-67.472283, -30.46747) (-67.311825, -30.637402) knots 0 0 0 0 1 1 1 1
  spline S39 degree 3 poles (-67.311825, -30.637402) (-66.144117, -31.875279) (-65.474369, -33.466544) (-65.474369, -35.003198) knots 0 0 0 0 1 1 1 1
  spline S40 degree 3 poles (-65.474369, -35.003198) (-65.474369, -35.235691) (-65.490092, -35.468184) (-65.521037, -35.69442) knots 0 0 0 0 1 1 1 1
  spline S41 degree 3 poles (-65.521037, -35.69442) (-65.662392, -36.727196) (-65.742203, -36.912345) (-65.886939, -37.248319) knots 0 0 0 0 1 1 1 1
  spline S42 degree 3 poles (-65.886939, -37.248319) (-65.95322, -37.402017) (-66.035394, -37.593252) (-66.140227, -37.905386) knots 0 0 0 0 1 1 1 1
  spline S43 degree 3 poles (-66.140227, -37.905386) (-66.187065, -38.045557) (-66.113343, -38.171528) (-65.983484, -38.195876) knots 0 0 0 0 1 1 1 1
  spline S44 degree 3 poles (-65.983484, -38.195876) (-65.671861, -38.254211) (-64.81121, -37.612698) (-64.607804, -37.088364) knots 0 0 0 0 1 1 1 1
  spline S45 degree 3 poles (-64.607804, -37.088364) (-64.421809, -36.609175) (-64.327627, -36.071651) (-64.327627, -35.49118) knots 0 0 0 0 1 1 1 1
  spline S46 degree 3 poles (-64.327627, -35.49118) (-64.327627, -34.885176) (-64.426541, -34.349342) (-64.498911, -33.958079) knots 0 0 0 0 1 1 1 1
  spline S47 degree 3 poles (-64.498911, -33.958079) (-64.532054, -33.779186) (-64.560966, -33.622105) (-64.566544, -33.525558) knots 0 0 0 0 1 1 1 1
  spline S48 degree 3 poles (-64.566544, -33.525558) (-64.345213, -33.511525) (-63.917426, -33.518455) (-63.609859, -33.52708) knots 0 0 0 0 1 1 1 1
  spline S49 degree 3 poles (-63.609859, -33.52708) (-63.490991, -35.795026) (-63.234488, -37.824564) (-62.835954, -39.62279) knots 0 0 0 0 1 1 1 1
  spline S50 degree 3 poles (-62.835954, -39.62279) (-63.599714, -40.892961) (-64.323742, -42.064727) (-64.45343, -42.183762) knots 0 0 0 0 1 1 1 1
  spline S51 degree 3 poles (-64.45343, -42.183762) (-64.530026, -42.240066) (-64.882398, -42.147071) (-65.139748, -42.079097) knots 0 0 0 0 1 1 1 1
  spline S52 degree 3 poles (-65.139748, -42.079097) (-65.459152, -41.994725) (-65.820993, -41.899359) (-66.199408, -41.876533) knots 0 0 0 0 1 1 1 1
  spline S53 degree 3 poles (-66.199408, -41.876533) (-66.709369, -41.845758) (-67.145783, -42.023975) (-67.335324, -42.202529) knots 0 0 0 0 1 1 1 1
  spline S54 degree 3 poles (-67.335324, -42.202529) (-67.420207, -42.282508) (-67.463155, -42.366881) (-67.463155, -42.453451) knots 0 0 0 0 1 1 1 1
  spline S55 degree 3 poles (-67.463155, -42.453451) (-67.463155, -42.513476) (-67.437452, -42.71063) (-67.105705, -42.730584) knots 0 0 0 0 1 1 1 1
  spline S56 degree 3 poles (-67.105705, -42.730584) (-66.618402, -42.759837) (-65.076, -43.454947) (-64.571111, -43.998727) knots 0 0 0 0 1 1 1 1
  spline S57 degree 3 poles (-64.571111, -43.998727) (-63.748, -44.885581) (-63.671914, -45.652724) (-63.715197, -46.806228) knots 0 0 0 0 1 1 1 1
  spline S58 degree 3 poles (-63.715197, -46.806228) (-63.750028, -47.737046) (-63.988104, -48.441795) (-64.10257, -48.780473) knots 0 0 0 0 1 1 1 1
  spline S59 degree 3 poles (-64.10257, -48.780473) (-64.151942, -48.926395) (-64.174429, -48.993011) (-64.174429, -49.049994) knots 0 0 0 0 1 1 1 1
  spline S60 degree 3 poles (-64.174429, -49.049994) (-64.174429, -49.117968) (-64.140951, -49.177825) (-64.084814, -49.209952) knots 0 0 0 0 1 1 1 1
  line L4 (-64.084814, -49.209952) -> (-63.984548, -49.255438)
  line L5 (-63.984548, -49.255438) -> (-63.900005, -49.206066)
  spline S61 degree 3 poles (-63.900005, -49.206066) (-63.701332, -49.090243) (-62.901725, -48.449236) (-62.620871, -47.429484) knots 0 0 0 0 1 1 1 1
  spline S62 degree 3 poles (-62.620871, -47.429484) (-62.458718, -46.840899) (-62.376541, -46.291876) (-62.376541, -45.797975) knots 0 0 0 0 1 1 1 1
  spline S63 degree 3 poles (-62.376541, -45.797975) (-62.376541, -44.846698) (-62.668891, -44.271299) (-62.882276, -43.851123) knots 0 0 0 0 1 1 1 1
  spline S64 degree 3 poles (-62.882276, -43.851123) (-62.999962, -43.619814) (-63.090254, -43.45022) (-63.064381, -43.31546) knots 0 0 0 0 1 1 1 1
  spline S65 degree 3 poles (-63.064381, -43.31546) (-63.026165, -43.119995) (-62.698309, -42.503171) (-62.264436, -41.749894) knots 0 0 0 0 1 1 1 1
  spline S66 degree 3 poles (-62.264436, -41.749894) (-61.523501, -44.056056) (-60.489711, -45.895878) (-59.153597, -47.29557) knots 0 0 0 0 1 1 1 1
  spline S67 degree 3 poles (-59.153597, -47.29557) (-52.388644, -54.38263) (-44.105134, -54.037188) (-38.338464, -52.499353) knots 0 0 0 0 1 1 1 1
  spline S68 degree 3 poles (-38.338464, -52.499353) (-36.767995, -52.080529) (-35.629373, -51.538607) (-34.798147, -51.143117) knots 0 0 0 0 1 1 1 1
  spline S69 degree 3 poles (-34.798147, -51.143117) (-33.036459, -50.304778) (-32.504854, -50.051825) (-31.274079, -52.30811) knots 0 0 0 0 1 1 1 1
extrude "Extrusion4" [suppressed]